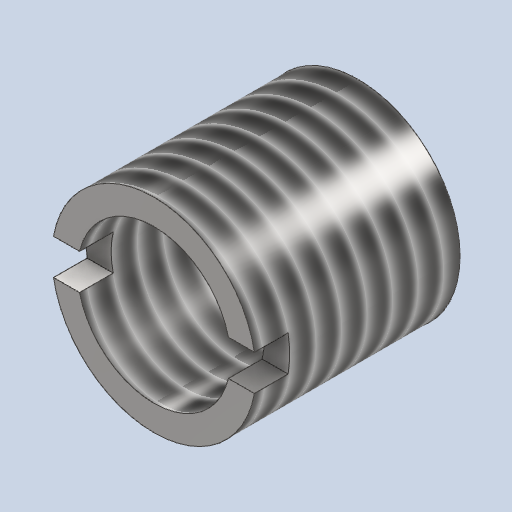
# Autodesk Inventor part: IRU-304S
Saved by Autodesk Inventor 2022.3 (Build 263350000, 350)
## iProperties
Part Number: IRU-304S
Material: ステンレス鋼 AISI 304
Document SubType Name: Modeling
Designer: Masato Kubotera
Density: 5.57467 g/cm^3
Appearance: 半つや出し
Catalog Web Link: https://www.hirosugi-net.co.jp/shop/g/g44607/
Description: ReadyMade
Mass: 0.12 g
Surface Area: 0.984466 cm^2
Volume: 0.0215259 cm^3
Author: Masato Kubotera
Autodesk Inventor part; units mm, degrees
ref_plane "YZ Plane" through (0, 0, 0) normal (1, 0, 0) x (0, 1, 0)
ref_plane "XZ Plane" through (0, 0, 0) normal (0, 1, 0) x (-1, 0, 0)
ref_plane "XY Plane" through (0, 0, 0) normal (0, 0, 1) x (1, 0, 0)
sketch "スケッチ1" plane through (0, 0, 0) normal (0, 0, 1) x (1, 0, 0)
  circle A0 centre (0, 0) radius 2
  circle A1 centre (0, 0) radius 1.5
  line L0 (-2, 0.35) -> (2, 0.35)
  line L1 (2, 0.35) -> (2, -0.35)
  line L2 (2, -0.35) -> (-2, -0.35)
  line L3 (-2, -0.35) -> (-2, 0.35)
  line L4 (-2, 0.35) -> (2, -0.35) construction
  line L5 (2, 0.35) -> (-2, -0.35) construction
  point P0 (1.4586, -0.35)
  point P1 (1.9691, -0.35)
  point P2 (1.9691, 0.35)
  point P3 (1.4586, 0.35)
  point P4 (-1.9691, -0.35)
  point P5 (-1.4586, -0.35)
  point P6 (-1.4586, 0.35)
  point P7 (-1.9691, 0.35)
  dimension "d0" = 4
  dimension "d1" = 3
  dimension "d8" = 0.7
  constraints: 12 end point, 2 centre point, 2 coincident, 2 midpoint, 2 parallel, 1 horizontal, 1 perpendicular, 1 tangent
  measures "d0" diameter of A0
  measures "d1" diameter of A1
  measures "d8" distance of L2.end L0.start
extrude "押し出し1" add sketch "スケッチ1" against normal blind 4 contours A0 L2 A1 L0 | L0 A1 A0 | A0 L2 A1 | L0 A1 L2 A0
thread "ねじ1" size "M3x0.5" class "6H" standard "ANSI Metric M Profile" full length
thread "ねじ2" size "M4x0.5" class "6g" standard "ANSI Metric M Profile" full length
extrude "押し出し2" cut sketch "スケッチ1" against normal blind 0.66 contours A0 L2 A1 L0 | L0 A1 L2 A0
